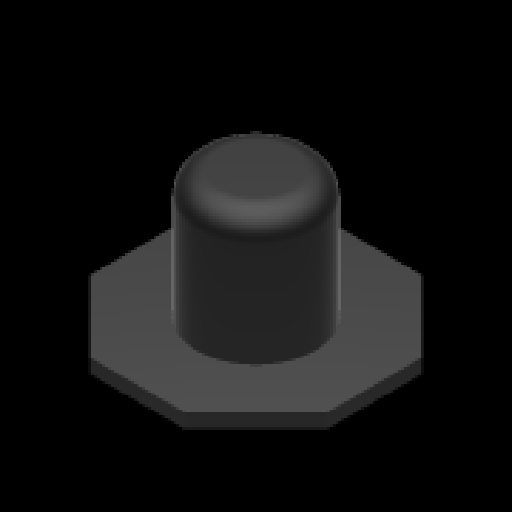
# Autodesk Inventor part: button
Saved by Autodesk Inventor 2024.4 (Build 284460000, 460)
## iProperties
Created: 2026-01-18
Part Number: button
Material: Ogólny
Document SubType Name: Modeling
Designer: User
Density: 1 g/cm^3
Appearance: Domyślna
Author: User
Autodesk Inventor part; units mm, degrees
ref_plane "YZ Plane" through (0, 0, 0) normal (1, 0, 0) x (0, 1, 0)
ref_plane "XZ Plane" through (0, 0, 0) normal (0, 1, 0) x (-1, 0, 0)
ref_plane "XY Plane" through (0, 0, 0) normal (0, 0, 1) x (1, 0, 0)
sketch "Szkic1" plane through (0, 0, 0) normal (0, 1, 0) x (-1, 0, 0)
  circle A0 centre (0, 0) radius 2.5
  line L0 (-5, 5) -> (5, 5)
  line L1 (5, 5) -> (5, -5)
  line L2 (5, -5) -> (-5, -5)
  line L3 (-5, -5) -> (-5, 5)
  line L4 (-5, 5) -> (5, -5) construction
  line L5 (5, 5) -> (-5, -5) construction
  circle A1 centre (0, 0) radius 2
  dimension "d0" = 5
  dimension "d1" = 10
  dimension "d2" = 10
  dimension "d7" = 4
  constraints: 12 end point, 2 centre point, 2 coincident, 2 midpoint, 2 parallel, 1 horizontal, 1 perpendicular
  measures "d0" diameter of A0
  measures "d1" distance of L1.end L2.end
  measures "d2" distance of L0.end L1.end
  measures "d7" diameter of A1
extrude "Wyciągnięcie proste1" add sketch "Szkic1" along normal blind 0.6 contours L0 L1 L2 L3
extrude "Wyciągnięcie proste2" add sketch "Szkic1" along normal blind 6 contours A0 | A1
extrude "Wyciągnięcie proste3" add sketch "Szkic1" against normal blind 0.4 contours A1
fillet "Zaokrąglenie1" radius 2 1 edges at (2, -0.4, 0)
chamfer "Faza1" distance 3 angle 45 4 edges at (-5, 0.3, 5) (5, 0.3, 5) (5, 0.3, -5) (-5, 0.3, -5)
fillet "Zaokrąglenie2" radius 1 1 edges at (2.5, 6, 0)
